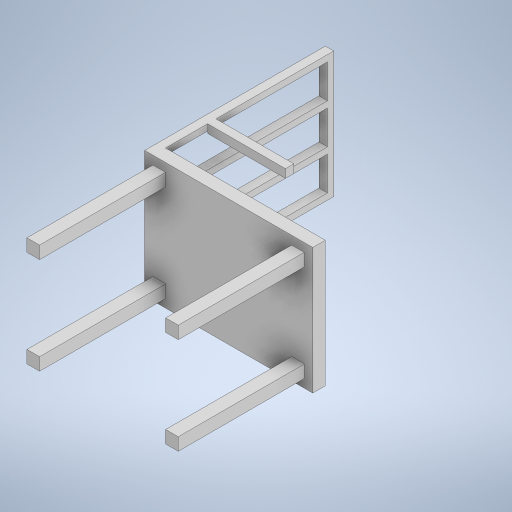
# Autodesk Inventor part: Maitri_chair
Saved by Autodesk Inventor 2023 (Build 270158000, 158)
## iProperties
Created: 2023-09-26
Part Number: Maitri_chair
Material: Generic
Document SubType Name: Modeling
Designer: maitr
Density: 1 g/cm^3
Appearance: Default
Author: maitr
Autodesk Inventor part; units mm, degrees
ref_plane "YZ Plane" through (0, 0, 0) normal (1, 0, 0) x (0, 1, 0)
ref_plane "XY Plane" through (0, 0, 0) normal (0, 0, 1) x (1, 0, 0)
sketch "Sketch1" plane through (0, 0, 0) normal (0, 0, 1) x (1, 0, 0)
  line L0 (0, 0) -> (400, 0)
  line L1 (400, 0) -> (400, 300)
  line L2 (400, 300) -> (0, 300)
  line L3 (0, 300) -> (0, 0)
  dimension "d0" = 400
  dimension "d1" = 300
  constraints: 8 end point, 2 parallel, 1 horizontal, 1 perpendicular
  measures "d0" distance of L2.end L1.end
  measures "d1" distance of L1.end L0.end
extrude "Extrusion1" add sketch "Sketch1" along normal blind 30
sketch "Sketch2" plane through (0, 0, 30) normal (0, 0, 1) x (1, 0, 0)
  line L0 (20, 280) -> (50, 280)
  line L1 (50, 280) -> (50, 250)
  line L2 (50, 250) -> (20, 250)
  line L3 (20, 250) -> (20, 280)
  line L4 (350, 280) -> (380, 280)
  line L5 (380, 280) -> (380, 250)
  line L6 (380, 250) -> (350, 250)
  line L7 (350, 250) -> (350, 280)
  line L8 (350, 20) -> (380, 20)
  line L9 (380, 20) -> (380, 50)
  line L10 (380, 50) -> (350, 50)
  line L11 (350, 50) -> (350, 20)
  line L12 (0, 300) -> (0, 0) projected
  line L13 (400, 300) -> (0, 300) projected
  line L14 (400, 0) -> (400, 300) projected
  line L15 (0, 0) -> (400, 0) projected
  line L16 (20, 50) -> (50, 50)
  line L17 (50, 50) -> (50, 20)
  line L18 (50, 20) -> (20, 20)
  line L19 (20, 20) -> (20, 50)
  dimension "d4" = 30
  dimension "d5" = 30
  dimension "d6" = 30
  dimension "d7" = 30
  dimension "d10" = 30
  dimension "d11" = 30
  dimension "d12" = 20
  dimension "d13" = 20
  dimension "d14" = 20
  dimension "d15" = 20
  dimension "d16" = 20
  dimension "d17" = 30
  dimension "d18" = 30
  dimension "d19" = 20
  dimension "d20" = 20
  constraints: 32 end point, 8 parallel, 4 horizontal, 4 perpendicular, 1 point on line
  measures "d4" distance of L1.end L2.end
  measures "d5" distance of L0.end L1.end
  measures "d6" distance of L5.end L6.end
  measures "d7" distance of L4.end L5.end
  measures "d10" distance of L10.end L9.end
  measures "d11" distance of L9.end L8.end
  measures "d12" distance between parallel lines of L12 L3
  measures "d13" distance between parallel lines of L13 L0
  measures "d14" distance between parallel lines of L14 L5
  measures "d15" distance between parallel lines of L14 L9
  measures "d16" distance between parallel lines of L15 L8
  measures "d17" distance of L17.end L18.end
  measures "d18" distance of L16.end L17.end
  measures "d19" distance between parallel lines of L15 L18
  measures "d20" distance between parallel lines of L12 L19
extrude "Extrusion2" add sketch "Sketch2" along normal blind 300 contours L0 L1 L2 L3 | L4 L5 L6 L7 | L11 L10 L9 L8 | L16 L17 L18 L19
sketch "Sketch3" plane through (0, 0, 0) normal (0, 0, -1) x (-1, 0, 0)
  line L0 (-400, 300) -> (0, 300) projected
  line L1 (0, 300) -> (-20, 300)
  line L2 (-20, 300) -> (-20, 285)
  line L3 (-20, 285) -> (0, 285)
  line L4 (0, 285) -> (0, 300)
  line L5 (0, 300) -> (0, 0) projected
  line L6 (-20, 20) -> (-50, 20) projected
  line L7 (0, 0) -> (-20, 0)
  line L8 (0, 190) -> (-20, 190)
  line L9 (-20, 190) -> (-20, 205)
  line L10 (-20, 205) -> (0, 205)
  line L11 (0, 205) -> (0, 190)
  line L12 (0, 110) -> (-20, 110)
  line L13 (-20, 110) -> (-20, 95)
  line L14 (-20, 95) -> (0, 95)
  line L15 (0, 95) -> (0, 110)
  line L16 (0, 0) -> (-20, 0)
  line L17 (-20, 0) -> (-20, 15)
  line L18 (-20, 15) -> (0, 15)
  line L19 (0, 15) -> (0, 0)
  point P0 (0, 95)
  point P1 (0, 205)
  dimension "d31" = 20
  dimension "d32" = 15
  dimension "d33" = 20
  dimension "d34" = 15
  dimension "d35" = 20
  dimension "d36" = 15
  dimension "d37" = 15
  dimension "d38" = 20
  dimension "d39" = 80
  dimension "d40" = 80
  dimension "d41" = 80
  constraints: 34 end point, 8 parallel, 5 horizontal, 4 perpendicular, 1 point on line
  measures "d31" distance of L2.end L3.end
  measures "d32" distance of L1.end L2.end
  measures "d33" distance of L8.start L8.end
  measures "d34" distance of L8.end L9.end
  measures "d35" distance of L13.end L14.end
  measures "d36" distance of L12.end L13.end
  measures "d37" distance of L16.end L17.end
  measures "d38" distance of L17.end L18.end
  measures "d39" distance of L10.end L3.end
  measures "d40" distance of L8.start L12.start
  measures "d41" distance of L14.end L18.end
extrude "Extrusion3" add sketch "Sketch3" along normal blind 385
sketch "Sketch4" plane through (0, 0, 0) normal (0, 1, 0) x (-1, 0, 0)
  line L0 (-20, 0) -> (-20, -385) projected
  line L1 (0, -400) -> (-20, -400)
  line L2 (-20, -400) -> (-20, -385)
  line L3 (-20, -385) -> (0, -385)
  line L4 (0, -385) -> (0, -400)
  point P0 (0, 0)
  dimension "d44" = 20
  dimension "d45" = 15
  constraints: 8 end point, 2 parallel, 1 horizontal, 1 perpendicular
  measures "d44" distance of L0.end L3.end
  measures "d45" distance of L1.end L0.end
extrude "Extrusion4" add sketch "Sketch4" along normal blind 300
sketch "Sketch5" plane through (0, 0, 0) normal (0, 1, 0) x (-1, 0, 0)
  line L0 (-20, 0) -> (-20, -385) projected
  line L1 (-20, -120) -> (-205, -120)
  line L2 (-205, -120) -> (-205, -100)
  line L3 (-205, -100) -> (-20, -100)
  line L4 (-20, -100) -> (-20, -120)
  line L5 (-400, 0) -> (-20, 0) projected
  point P0 (0, 0)
  point P1 (-20, -100)
  dimension "d48" = 185
  dimension "d49" = 20
  dimension "d50" = 100
  constraints: 8 end point, 2 parallel, 1 horizontal, 1 perpendicular, 1 point on line
  measures "d48" distance of L2.end L3.end
  measures "d49" distance of L1.end L2.end
  measures "d50" distance between parallel lines of L3 L5
ref_plane "Work Plane1" through (0, 150, 0) normal (0, 1, 0) x (-1, 0, 0)
extrude "Extrusion5" add sketch "Sketch5" along normal blind 20
mirror "Mirror1" about plane through (0, 150, 0) normal (0, 1, 0) of "Extrusion5"
body "Solid1"
